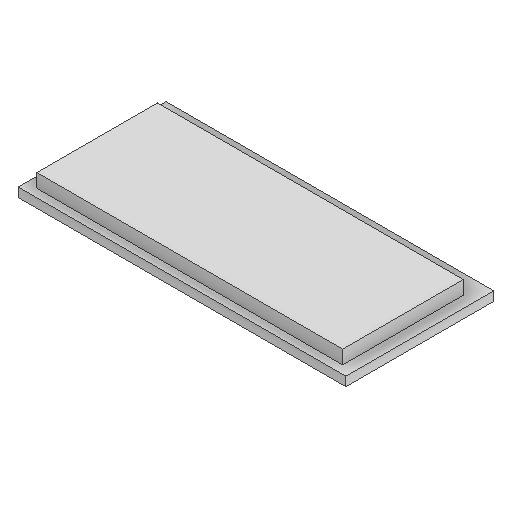
# Autodesk Inventor part: Base Box Lid
Saved by Autodesk Inventor 2025.1 (Build 291241020, 241B)
## iProperties
Created: 2025-01-03
Part Number: Base Box Lid
Material: Generic
Document SubType Name: Modeling
Designer: alexa
Density: 1 g/cm^3
Appearance: Default
Author: alexa
Autodesk Inventor part; units mm, degrees
ref_plane "YZ Plane" through (0, 0, 0) normal (1, 0, 0) x (0, 1, 0)
ref_plane "XZ Plane" through (0, 0, 0) normal (0, 1, 0) x (-1, 0, 0)
ref_plane "XY Plane" through (0, 0, 0) normal (0, 0, 1) x (1, 0, 0)
sketch "Sketch1" plane through (0, 0, 0) normal (0, 1, 0) x (-1, 0, 0)
  line L0 (0, 0) -> (-182.88, 0)
  line L1 (-182.88, 0) -> (-182.88, -82.55)
  line L2 (-182.88, -82.55) -> (0, -82.55)
  line L3 (0, -82.55) -> (0, 0)
  dimension "d0" = 82.55
  dimension "d1" = 182.88
  constraints: 8 end point, 2 parallel, 1 horizontal, 1 perpendicular
  measures "d0" distance of L2.end L0.start
  measures "d1" distance of L1.end L2.end
extrude "Extrusion1" add sketch "Sketch1" along normal blind 5.08
sketch "Sketch2" plane through (0, 5.08, 0) normal (0, 1, 0) x (1, 0, 0)
  line L0 (5.842, 71.882) -> (176.53, 71.882)
  line L1 (176.53, 71.882) -> (176.53, 4.572)
  line L2 (176.53, 4.572) -> (5.842, 4.572)
  line L3 (5.842, 4.572) -> (5.842, 71.882)
  line L4 (0, 82.55) -> (0, 0) projected
  line L5 (182.88, 0) -> (182.88, 82.55) projected
  line L6 (0, 0) -> (182.88, 0) projected
  line L7 (182.88, 82.55) -> (0, 82.55) projected
  line L8 (172.232, 67.584) -> (10.14, 67.584)
  line L9 (10.14, 67.584) -> (10.14, 8.87)
  line L10 (10.14, 8.87) -> (172.232, 8.87)
  line L11 (172.232, 8.87) -> (172.232, 67.584)
  point P0 (182.88, 41.275)
  dimension "d4" = 5.842
  dimension "d5" = 6.35
  dimension "d6" = 4.572
  dimension "d7" = 10.668
  constraints: 16 end point, 4 parallel, 2 perpendicular, 1 horizontal, 1 midpoint, 3 other
  measures "d4" distance between parallel lines of L4 L3
  measures "d5" distance from line of point (182.88, 41.275) L1
  measures "d6" distance between parallel lines of L2 L6
  measures "d7" distance between parallel lines of L0 L7
extrude "Extrusion2" add sketch "Sketch2" along normal blind 7.62 contours L0 L1 L2 L3 | L11 L10 L9 L8
sketch "Sketch3" plane through (0, 0, 0) normal (0, -1, 0) x (1, 0, 0)
  line L0 (97.536, -57.277) -> (85.344, -57.277)
  line L1 (85.344, -57.277) -> (85.344, -25.273)
  line L2 (85.344, -25.273) -> (97.536, -25.273)
  line L3 (97.536, -25.273) -> (97.536, -57.277)
  line L4 (182.88, 0) -> (182.88, -82.55) projected
  line L5 (0, 0) -> (182.88, 0) projected
  line L6 (85.344, -43.307) -> (59.944, -43.307)
  line L7 (59.944, -43.307) -> (59.944, -39.243)
  line L8 (59.944, -39.243) -> (85.344, -39.243)
  line L9 (85.344, -39.243) -> (85.344, -43.307)
  point P0 (97.536, -41.275)
  point P1 (182.88, -41.275)
  point P2 (91.44, -25.273)
  point P3 (91.44, 0)
  point P4 (59.944, -41.275)
  point P5 (85.344, -41.275)
  dimension "d10" = 32.004
  dimension "d11" = 12.192
  dimension "d12" = 25.4
  dimension "d13" = 4.064
  constraints: 16 end point, 6 midpoint, 4 parallel, 2 horizontal, 2 horizontal alignment, 2 perpendicular, 1 point on line, 1 vertical alignment
  measures "d10" distance of L2.end L0.start
  measures "d11" distance of L0.start L0.end
  measures "d12" distance of L6.start L6.end
  measures "d13" distance of L6.end L7.end
extrude "Extrusion3" add sketch "Sketch3" along normal blind 6.35
sketch "Sketch4" plane through (0, -6.35, 0) normal (0, -1, 0) x (1, 0, 0)
  line L0 (97.282, -52.197) -> (85.598, -52.197)
  line L1 (85.598, -52.197) -> (85.598, -30.353)
  line L2 (85.598, -30.353) -> (97.282, -30.353)
  line L3 (97.282, -30.353) -> (97.282, -52.197)
  line L4 (97.536, -57.277) -> (97.536, -25.273) projected
  line L5 (85.344, -57.277) -> (97.536, -57.277) projected
  point P0 (0, 0)
  point P1 (85.598, -41.275)
  point P2 (97.536, -41.275)
  point P3 (91.44, -52.197)
  point P4 (91.44, -57.277)
  dimension "d16" = 21.844
  dimension "d17" = 11.684
  constraints: 8 end point, 4 midpoint, 2 parallel, 1 horizontal, 1 horizontal alignment, 1 perpendicular, 1 vertical alignment
  measures "d16" distance of L0.end L1.end
  measures "d17" distance between parallel lines of L1 L3
extrude "Extrusion4" add sketch "Sketch4" along normal blind 12.7
body "Solid1"
